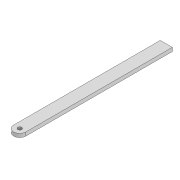
# Autodesk Inventor part: Part_2_p1
Saved by Autodesk Inventor 2022 (Build 260153000, 153)
## iProperties
Created: 2022-04-22
Part Number: Part_2_p1
Material: Generic
Document SubType Name: Modeling
Designer: dell
Density: 1 g/cm^3
Appearance: Default
Mass: 2.94792 g
Surface Area: 26.4711 cm^2
Volume: 2.94792 cm^3
Author: dell
Autodesk Inventor part; units mm, degrees
ref_plane "YZ Plane" through (0, 0, 0) normal (1, 0, 0) x (0, 1, 0)
ref_plane "XZ Plane" through (0, 0, 0) normal (0, 1, 0) x (-1, 0, 0)
ref_plane "XY Plane" through (0, 0, 0) normal (0, 0, 1) x (1, 0, 0)
sketch "Sketch1" plane through (0, 0, 0) normal (0, 1, 0) x (-1, 0, 0)
  line L0 (0, 0) -> (0, -261.6) construction
  line L1 (5, 0) -> (5, -261.6)
  line L2 (-5, -261.6) -> (-5, 0)
  arc A0 (5, 0) -> (-5, 0) centre (0, 0) ccw
  arc A1 (-5, -261.6) -> (5, -261.6) centre (0, -261.6) ccw
  circle A2 centre (0, 0) radius 1.65
  circle A3 centre (0, -261.6) radius 1.65
  circle A4 centre (0, -153.559) radius 1.65
  point P0 (0, -130.8)
  dimension "d0" = 3.3
  dimension "d1" = 3.3
  dimension "d2" = 10
  dimension "d3" = 261.6
  dimension "d4" = 3.3
  dimension "d5" = 153.559
  constraints: 8 end point, 5 centre point, 4 point on circle, 4 tangent, 2 coincident, 1 midpoint, 1 parallel, 1 point on line, 1 vertical
  measures "d0" diameter of A2
  measures "d1" diameter of A3
  measures "d2" distance between parallel lines of L2 L1
  measures "d3" distance of L0.end L0.start
  measures "d4" diameter of A4
  measures "d5" distance of L0.start A4.centre
extrude "Extrusion1" add sketch "Sketch1" along normal blind 3
sketch "Sketch3" plane through (0, 3, 0) normal (0, 1, 0) x (1, 0, 0)
  line L0 (-22.4574, 275.926) -> (26.2563, 275.926)
  line L1 (26.2563, 275.926) -> (26.2563, 121.3008)
  line L2 (26.2563, 121.3008) -> (-22.4574, 121.3008)
  line L3 (-22.4574, 121.3008) -> (-22.4574, 275.926)
  line L4 (-103.4002, 357.0257) -> (155.5228, 357.0257)
  line L5 (155.5228, 357.0257) -> (155.5228, -67.8162)
  line L6 (155.5228, -67.8162) -> (-103.4002, -67.8162)
  line L7 (-103.4002, -67.8162) -> (-103.4002, 357.0257)
  point P0 (0, 0)
  constraints: 16 end point, 4 parallel, 2 horizontal, 2 perpendicular
extrude "Extrusion2" cut sketch "Sketch3" against normal blind 100 contours L0 L1 L2 L3
body "Solid1"
